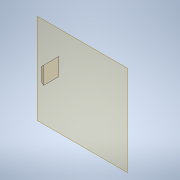
# Autodesk Inventor part: 20_Cube_Inser_Flexuremanipulator_springlock_v3
Saved by Autodesk Inventor 2022.3 (Build 263350000, 350)
## iProperties
Created: 2021-12-17
Part Number: 20_Cube_Inser_Flexuremanipulator_springlock_v3
Material: Generisch
Document SubType Name: Modeling
Designer: diederichbenedict
Density: 1 g/cm^3
Appearance: Vorgabe
Author: diederichbenedict
Autodesk Inventor part; units mm, degrees
ref_plane "YZ Plane" through (0, 0, 0) normal (1, 0, 0) x (0, 1, 0)
ref_plane "XZ Plane" through (0, 0, 0) normal (0, 1, 0) x (-1, 0, 0)
ref_plane "XY Plane" through (0, 0, 0) normal (0, 0, 1) x (1, 0, 0)
ref_plane "Arbeitsebene1" through (0, 0, 0) normal (0, 0, 1) x (1, 0, 0)
sketch "Skizze1" plane through (0, 0, 0) normal (0, 0, 1) x (1, 0, 0)
  line L0 (-23.1578, -6.2841) -> (-24.6578, -4.7841) projected
  line L1 (-24.6578, -4.7841) -> (-12.6578, -4.7841) projected
  line L2 (-12.6578, -4.7841) -> (-14.1578, -6.2841) projected
  line L3 (-14.1578, -6.2841) -> (-23.1578, -6.2841) projected
  line L4 (-43.426, 23.1477) -> (-41.926, 24.6477) projected
  line L5 (-41.926, 24.6477) -> (-41.926, 12.6477) projected
  line L6 (-41.926, 12.6477) -> (-43.426, 14.1477) projected
  line L7 (-43.426, 14.1477) -> (-43.426, 1.4359) projected
  line L8 (-43.426, 1.4359) -> (-39.726, 1.4359) projected
  line L9 (-39.726, 1.4359) -> (-35.546, -2.7441) projected
  line L10 (-35.546, -2.7441) -> (-35.546, -6.4241) projected
  line L11 (-35.546, -6.4241) -> (-1.606, -6.4241) projected
  line L12 (-1.606, -6.4241) -> (-1.606, -2.7441) projected
  line L13 (-1.606, -2.7441) -> (2.574, 1.4359) projected
  line L14 (2.574, 1.4359) -> (6.414, 1.4359) projected
  line L15 (6.414, 1.4359) -> (6.414, 10.6477) projected
  line L16 (6.414, 10.6477) -> (10.414, 10.6477) projected
  line L17 (10.414, 26.6477) -> (10.414, 10.6477) projected
  line L18 (6.414, 26.6477) -> (10.414, 26.6477) projected
  line L19 (6.414, 26.6477) -> (6.414, 35.5359) projected
  line L20 (6.414, 35.5359) -> (2.574, 35.5359) projected
  line L21 (2.574, 35.5359) -> (-1.606, 39.7429) projected
  line L22 (-1.606, 39.7429) -> (-1.606, 43.5559) projected
  line L23 (-1.606, 43.5559) -> (-9.6578, 43.5559) projected
  line L24 (-9.6578, 43.5559) -> (-9.6578, 47.5559) projected
  line L25 (-27.6578, 47.5559) -> (-9.6578, 47.5559) projected
  line L26 (-27.6578, 43.5559) -> (-27.6578, 47.5559) projected
  line L27 (-27.6578, 43.5559) -> (-32.737, 43.5559) projected
  line L28 (-32.737, 43.5559) -> (-35.546, 43.5359) projected
  line L29 (-35.546, 43.5359) -> (-35.519, 39.7429) projected
  line L30 (-35.519, 39.7429) -> (-39.726, 35.5359) projected
  line L31 (-39.726, 35.5359) -> (-43.426, 35.5359) projected
  line L32 (-43.426, 35.5359) -> (-43.426, 23.1477) projected
  line L33 (-3.1655, 23.9804) -> (-4.415, 22.7309) projected
  line L34 (-4.415, 22.7309) -> (-4.415, 14.4009) projected
  line L35 (-4.415, 14.4009) -> (-3.1655, 13.1514) projected
  line L36 (-3.1655, 13.1514) -> (-3.1655, 9.27) projected
  line L37 (-3.1655, 9.27) -> (-8.0306, 4.4049) projected
  line L38 (-8.0306, 4.4049) -> (-27.8429, 4.4049) projected
  line L39 (-27.8429, 4.4049) -> (-33.1694, 9.7314) projected
  line L40 (-33.1694, 9.7314) -> (-33.1694, 13.1514) projected
  line L41 (-33.1694, 13.1514) -> (-31.9199, 14.4009) projected
  line L42 (-31.9199, 14.4009) -> (-31.9199, 22.7309) projected
  line L43 (-31.9199, 22.7309) -> (-33.1694, 23.9804) projected
  line L44 (-33.1694, 23.9804) -> (-33.1694, 26.7231) projected
  arc A0 (-31.9199, 26.7231) -> (-33.1694, 26.7231) centre (-32.5446, 26.7231) ccw projected
  line L45 (-31.9199, 26.7231) -> (-31.9199, 23.9804) projected
  line L46 (-31.9199, 23.9804) -> (-30.6704, 22.7309) projected
  line L47 (-30.6704, 22.7309) -> (-30.6704, 14.4009) projected
  line L48 (-30.6704, 14.4009) -> (-31.9199, 13.1514) projected
  line L49 (-31.9199, 13.1514) -> (-31.9199, 9.7314) projected
  line L50 (-31.9199, 9.7314) -> (-27.0099, 4.8214) projected
  line L51 (-27.0099, 4.8214) -> (-8.8636, 4.8214) projected
  line L52 (-8.8636, 4.8214) -> (-4.415, 9.27) projected
  line L53 (-4.415, 9.27) -> (-4.415, 13.1514) projected
  line L54 (-4.415, 13.1514) -> (-5.6645, 14.4009) projected
  line L55 (-5.6645, 14.4009) -> (-5.6645, 22.7309) projected
  line L56 (-5.6645, 22.7309) -> (-4.415, 23.9804) projected
  line L57 (-4.415, 23.9804) -> (-4.415, 27.27) projected
  arc A1 (-3.1655, 27.27) -> (-4.415, 27.27) centre (-3.7903, 27.27) ccw projected
  line L58 (-3.1655, 27.27) -> (-3.1655, 23.9804) projected
  line L59 (-1.083, 22.7309) -> (-2.3325, 23.9804) projected
  line L60 (-2.3325, 23.9804) -> (-2.3325, 27.7462) projected
  line L61 (-2.3325, 27.7462) -> (-6.8967, 32.3104) projected
  line L62 (-6.8967, 32.3104) -> (-29.2772, 32.3104) projected
  line L63 (-29.2772, 32.3104) -> (-34.0024, 27.5852) projected
  line L64 (-34.0024, 27.5852) -> (-34.0024, 23.9804) projected
  line L65 (-34.0024, 23.9804) -> (-35.2519, 22.7309) projected
  line L66 (-35.2519, 22.7309) -> (-35.2519, 14.4009) projected
  line L67 (-35.2519, 14.4009) -> (-34.0024, 13.1514) projected
  line L68 (-34.0024, 13.1514) -> (-34.0024, 9.1062) projected
  arc A2 (-35.2519, 9.1062) -> (-34.0024, 9.1062) centre (-34.6271, 9.1062) ccw projected
  line L69 (-35.2519, 9.1062) -> (-35.2519, 13.1514) projected
  line L70 (-35.2519, 13.1514) -> (-36.5014, 14.4009) projected
  line L71 (-36.5014, 14.4009) -> (-36.5014, 22.7309) projected
  line L72 (-36.5014, 22.7309) -> (-35.2519, 23.9804) projected
  line L73 (-35.2519, 23.9804) -> (-35.2519, 27.5118) projected
  line L74 (-35.2519, 27.5118) -> (-30.0368, 32.7269) projected
  line L75 (-30.0368, 32.7269) -> (-6.0637, 32.7269) projected
  line L76 (-6.0637, 32.7269) -> (-1.083, 27.7462) projected
  line L77 (-1.083, 27.7462) -> (-1.083, 23.9804) projected
  line L78 (-1.083, 23.9804) -> (0.1665, 22.7309) projected
  line L79 (0.1665, 22.7309) -> (0.1665, 14.4009) projected
  line L80 (0.1665, 14.4009) -> (-1.083, 13.1514) projected
  line L81 (-1.083, 13.1514) -> (-1.083, 9.9845) projected
  line L82 (-1.083, 9.9845) -> (-0.1206, 9.9845) projected
  arc A3 (0.6639, 9.2286) -> (-0.1206, 9.9845) centre (0.6639, 10.0136) ccw projected
  line L83 (0.6639, 9.2286) -> (-2.3325, 9.2286) projected
  line L84 (-2.3325, 9.2286) -> (-2.3325, 13.1514) projected
  line L85 (-2.3325, 13.1514) -> (-1.083, 14.4009) projected
  line L86 (-1.083, 14.4009) -> (-1.083, 22.7309) projected
  line L87 (-7.8034, -0.5931) -> (-11.8361, -0.5931) projected
  line L88 (-11.8361, -0.5931) -> (-13.0856, 0.6564) projected
  line L89 (-13.0856, 0.6564) -> (-23.0816, 0.6564) projected
  line L90 (-23.0816, 0.6564) -> (-24.3311, -0.5931) projected
  line L91 (-24.3311, -0.5931) -> (-29.5122, -0.5931) projected
  arc A4 (-29.5122, 0.6564) -> (-29.5122, -0.5931) centre (-29.5122, 0.0317) ccw projected
  line L92 (-29.5122, 0.6564) -> (-24.3311, 0.6564) projected
  line L93 (-24.3311, 0.6564) -> (-23.0816, 1.9059) projected
  line L94 (-23.0816, 1.9059) -> (-13.0856, 1.9059) projected
  line L95 (-13.0856, 1.9059) -> (-11.8361, 0.6564) projected
  line L96 (-11.8361, 0.6564) -> (-7.8034, 0.6564) projected
  line L97 (-7.8034, 0.6564) -> (-0.25, 8.2098) projected
  line L98 (-0.25, 8.2098) -> (3.4985, 8.2098) projected
  line L99 (3.4985, 8.2098) -> (3.4985, 28.6211) projected
  line L100 (3.4985, 28.6211) -> (0.051, 28.6211) projected
  line L101 (0.051, 28.6211) -> (-7.8034, 36.4754) projected
  line L102 (-7.8034, 36.4754) -> (-11.8361, 36.4754) projected
  line L103 (-11.8361, 36.4754) -> (-13.0856, 35.2259) projected
  line L104 (-13.0856, 35.2259) -> (-23.0816, 35.2259) projected
  line L105 (-23.0816, 35.2259) -> (-24.3311, 36.4754) projected
  line L106 (-24.3311, 36.4754) -> (-27.1009, 36.4754) projected
  arc A5 (-28.3504, 37.7249) -> (-27.1009, 36.4754) centre (-28.3504, 36.4754) ccw projected
  line L107 (-28.3504, 37.7249) -> (-24.3311, 37.7249) projected
  line L108 (-24.3311, 37.7249) -> (-23.0816, 36.4754) projected
  line L109 (-23.0816, 36.4754) -> (-13.0856, 36.4754) projected
  line L110 (-13.0856, 36.4754) -> (-11.8361, 37.7249) projected
  line L111 (-11.8361, 37.7249) -> (-7.8034, 37.7249) projected
  line L112 (-7.8034, 37.7249) -> (0.051, 29.8706) projected
  line L113 (0.051, 29.8706) -> (3.915, 29.8706) projected
  line L114 (3.915, 29.8706) -> (3.915, 6.9603) projected
  line L115 (3.915, 6.9603) -> (-0.25, 6.9603) projected
  line L116 (-0.25, 6.9603) -> (-7.8034, -0.5931) projected
  arc A6 (-31.6721, -1.088) -> (-30.301, -2.6756) centre (-30.301, -1.2897) ccw projected
  line L117 (-31.6721, -1.088) -> (-31.6721, 1.5931) projected
  line L118 (-31.6721, 1.5931) -> (-37.9016, 7.8227) projected
  line L119 (-37.9016, 7.8227) -> (-37.9016, 29.3992) projected
  line L120 (-37.9016, 29.3992) -> (-31.6721, 35.6287) projected
  line L121 (-31.6721, 35.6287) -> (-31.6721, 36.973) projected
  arc A7 (-29.7485, 39.8074) -> (-31.6721, 36.973) centre (-28.6221, 36.973) ccw projected
  line L122 (-29.7485, 39.8074) -> (-24.3311, 39.8074) projected
  line L123 (-24.3311, 39.8074) -> (-23.0816, 41.0569) projected
  line L124 (-23.0816, 41.0569) -> (-13.0856, 41.0569) projected
  line L125 (-13.0856, 41.0569) -> (-11.8361, 39.8074) projected
  line L126 (-11.8361, 39.8074) -> (-6.9454, 39.8074) projected
  arc A8 (-6.9454, 38.5579) -> (-6.9454, 39.8074) centre (-6.9454, 39.1827) ccw projected
  line L127 (-6.9454, 38.5579) -> (-11.8361, 38.5579) projected
  line L128 (-11.8361, 38.5579) -> (-13.0856, 39.8074) projected
  line L129 (-13.0856, 39.8074) -> (-23.0816, 39.8074) projected
  line L130 (-23.0816, 39.8074) -> (-24.3311, 38.5579) projected
  line L131 (-24.3311, 38.5579) -> (-28.5767, 38.5579) projected
  arc A9 (-28.5767, 38.5579) -> (-31.2556, 36.5303) centre (-28.5767, 35.7744) ccw projected
  line L132 (-31.2556, 36.5303) -> (-31.2556, 34.3792) projected
  line L133 (-31.2556, 34.3792) -> (-37.4851, 28.1497) projected
  line L134 (-37.4851, 28.1497) -> (-37.4851, 9.0722) projected
  line L135 (-37.4851, 9.0722) -> (-31.2556, 2.8426) projected
  line L136 (-31.2556, 2.8426) -> (-31.2556, -0.2985) projected
  arc A10 (-31.2556, -0.2985) -> (-30.128, -1.4261) centre (-30.128, -0.2985) ccw projected
  line L137 (-30.128, -1.4261) -> (-24.3311, -1.4261) projected
  line L138 (-24.3311, -1.4261) -> (-23.0816, -2.6756) projected
  line L139 (-23.0816, -2.6756) -> (-13.0856, -2.6756) projected
  line L140 (-13.0856, -2.6756) -> (-11.8361, -1.4261) projected
  line L141 (-11.8361, -1.4261) -> (-8.1549, -1.4261) projected
  arc A11 (-9.4975, -2.7687) -> (-8.1549, -1.4261) centre (-8.1549, -2.7687) ccw projected
  line L142 (-9.4975, -2.7687) -> (-9.4975, -2.6756) projected
  line L143 (-9.4975, -2.6756) -> (-11.8361, -2.6756) projected
  line L144 (-11.8361, -2.6756) -> (-13.0856, -3.9251) projected
  line L145 (-13.0856, -3.9251) -> (-23.0816, -3.9251) projected
  line L146 (-23.0816, -3.9251) -> (-24.3311, -2.6756) projected
  line L147 (-24.3311, -2.6756) -> (-30.301, -2.6756) projected
  spline S0 degree 3 poles (-22.5816, 9.4578) (-23.782, 9.9576) (-24.8728, 10.6879) (-26.7215, 12.5314) (-27.459, 13.6295) (-28.4771, 16.0552) (-28.7445, 17.3609) (-28.7639, 19.7945) (-28.5901, 20.9017) (-27.8908, 23.023) (-27.368, 24.0222) (-26.6946, 24.9175) knots 0 0 0 0 0.390087 0.390087 0.7831 0.7831 1.17904 1.17904 1.512851 1.512851 1.848728 1.848728 1.848728 1.848728 projected
  arc A12 (-14.4263, 28.0017) -> (-26.6946, 24.9175) centre (-18.576, 18.5659) ccw projected
  spline S1 degree 3 poles (-14.4263, 28.0017) (-13.2128, 27.4401) (-12.1202, 26.6478) (-10.3081, 24.6948) (-9.6034, 23.5555) (-8.6755, 21.0795) (-8.4577, 19.7679) (-8.5322, 17.3567) (-8.7442, 16.2748) (-9.5078, 14.2292) (-10.0521, 13.2785) (-10.7394, 12.4349) knots 0 0 0 0 0.401148 0.401148 0.799369 0.799369 1.194661 1.194661 1.523406 1.523406 1.850084 1.850084 1.850084 1.850084 projected
  arc A13 (-22.5816, 9.4578) -> (-10.7394, 12.4349) centre (-18.576, 18.5659) ccw projected
  circle A14 centre (-8.9594, 8.9493) radius 0.9 projected
  circle A15 centre (-28.1927, 28.1826) radius 0.9 projected
  circle A16 centre (7.1645, 15.1129) radius 1.45 projected
  circle A17 centre (-22.1312, 44.3064) radius 1.45 projected
  circle A18 centre (-14.8592, 44.3064) radius 1.45 projected
  circle A19 centre (7.1645, 22.3009) radius 1.45 projected
  circle A20 centre (-28.1927, 8.9493) radius 0.9 projected
  circle A21 centre (-8.9594, 28.1826) radius 0.9 projected
  line L148 (-42.026, 12.8892) -> (-42.026, 24.4063) construction
  line L149 (-42.026, 24.4063) -> (-43.526, 22.9063) construction
  line L150 (-43.526, 22.9063) -> (-43.526, 35.6359) construction
  line L151 (-43.526, 35.6359) -> (-39.7675, 35.6359) construction
  line L152 (-39.7675, 35.6359) -> (-35.6193, 39.784) construction
  line L153 (-35.6193, 39.784) -> (-35.6467, 43.6352) construction
  line L154 (-35.6467, 43.6352) -> (-32.7374, 43.6559) construction
  line L155 (-32.7374, 43.6559) -> (-27.7578, 43.6559) construction
  line L156 (-27.7578, 43.6559) -> (-27.7578, 47.6559) construction
  line L157 (-27.7578, 47.6559) -> (-9.5578, 47.6559) construction
  line L158 (-9.5578, 47.6559) -> (-9.5578, 43.6559) construction
  line L159 (-9.5578, 43.6559) -> (-1.506, 43.6559) construction
  line L160 (-1.506, 43.6559) -> (-1.506, 39.7842) construction
  line L161 (-1.506, 39.7842) -> (2.6156, 35.6359) construction
  line L162 (2.6156, 35.6359) -> (6.514, 35.6359) construction
  line L163 (6.514, 35.6359) -> (6.514, 26.7477) construction
  line L164 (6.514, 26.7477) -> (10.514, 26.7477) construction
  line L165 (10.514, 26.7477) -> (10.514, 10.5477) construction
  line L166 (10.514, 10.5477) -> (6.514, 10.5477) construction
  line L167 (6.514, 10.5477) -> (6.514, 1.3359) construction
  line L168 (6.514, 1.3359) -> (2.6154, 1.3359) construction
  line L169 (2.6154, 1.3359) -> (-1.506, -2.7855) construction
  line L170 (-1.506, -2.7855) -> (-1.506, -6.5241) construction
  line L171 (-1.506, -6.5241) -> (-35.646, -6.5241) construction
  line L172 (-35.646, -6.5241) -> (-35.646, -2.7855) construction
  line L173 (-35.646, -2.7855) -> (-39.7675, 1.3359) construction
  line L174 (-39.7675, 1.3359) -> (-43.526, 1.3359) construction
  line L175 (-43.526, 1.3359) -> (-43.526, 14.3892) construction
  line L176 (-43.526, 14.3892) -> (-42.026, 12.8892) construction
  line L177 (-42.026, 12.8892) -> (-43.426, 14.2892)
  line L178 (-42.026, 12.8892) -> (-42.026, 24.4063)
  line L179 (-42.026, 24.4063) -> (-43.426, 23.0063)
  line L180 (-43.426, 23.0063) -> (-43.426, 14.2892)
  point P0 (0, 0)
  dimension "d0" = 0.1
  constraints: 66 end point, 2 collinear, 1 parallel, 1 point on line, 28 other
  measures "d0" distance between parallel lines of L5 L148
extrude "Extrusion1" add sketch "Skizze1" against normal blind 10 contours L177 L180 L179 L178
